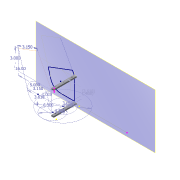
# Autodesk Inventor part: TransferChute
Saved by Autodesk Inventor 2018 (Build 220112000, 112)
## iProperties
Created: 2018-12-12
Part Number: TransferChute
Material: Generic
Document SubType Name: Modeling
Designer: ball
Density: 1 g/cm^3
Appearance: Default
Author: ball
Autodesk Inventor part; units mm, degrees
ref_plane "YZ Plane" through (0, 0, 0) normal (1, 0, 0) x (0, 1, 0)
ref_plane "XZ Plane" through (0, 0, 0) normal (0, 1, 0) x (-1, 0, 0)
sketch "Sketch1" plane through (0, 0, 0) normal (0, 0, 1) x (1, 0, 0)
  line L0 (-8, 88) -> (-8, 100) construction
  line L1 (272, 92) -> (-8, 92) construction
  line L2 (272, 92) -> (-8, 92) construction
  line L3 (-8, 88) -> (-8, 100) construction
  line L4 (-20, 88) -> (-20, 90.5) construction
  line L5 (-8, 88) -> (-20, 88) construction
  line L6 (-20, 88) -> (-20, 8) construction
  line L7 (-20, 88) -> (-147, 88) construction
  line L8 (-147, 88) -> (-147, 164.2) construction
  line L9 (-147, 164.2) -> (-72.1492, 192.4658) construction
  line L10 (-72.1492, 192.4658) -> (-20, 88) construction
  line L11 (-20, 48) -> (-111.8972, 48) construction
  circle A0 centre (-72.0661, 48) radius 40.005 construction
  line L12 (-71.4336, 8) -> (-20, 8) construction
  line L13 (-147, 164.2) -> (-110.5216, 36.974) construction
  point P0 (0, 0)
  dimension "d21" = 80.01
  dimension "d4" = 127
  dimension "d5" = 76.2
  dimension "d6" = 80.01
  dimension "d20" = 91.8972
  dimension "d23" = 15.999
  constraints: 24 end point, 5 horizontal, 4 vertical, 1 coincident, 1 midpoint, 1 point on line, 11 other
  measures "d4" distance of L7.start L7.end
  measures "d5" distance of L7.end L8.end
  measures "d6" distance of L8.end L9.end
  measures "d20" distance of L11.start L11.end
  measures "d23" angle of L8 L13
sketch "Sketch2" plane through (0, 0, 0) normal (0, 1, 0) x (-1, 0, 0)
  line L0 (10.5, -88) -> (20, -88) construction
  circle A0 centre (16, -84) radius 2 construction
  line L1 (16, -84) -> (31.875, -56.5037) construction
  line L2 (16, -84) -> (47.75, -84) construction
  line L3 (20, -88) -> (20, 0) construction
  line L4 (31.875, -56.5037) -> (31.875, -16.4987) construction
  circle A1 centre (31.875, -16.4987) radius 40.005 construction
  circle A2 centre (31.875, -56.5037) radius 40.005 construction
  circle A3 centre (31.875, -56.5037) radius 80.01 construction
  line L5 (111.885, -52.8947) -> (111.885, -78.2947) construction
  point P0 (0, 0)
  dimension "d10" = 31.75
  dimension "d11" = 60
  dimension "d13" = 40.005
  dimension "d14" = 80.01
  dimension "d15" = 80.01
  dimension "d17" = 160.02
  dimension "d18" = 11.875
  dimension "d24" = 25.4
  dimension "d25" = 91.885
  constraints: 12 end point, 4 centre point, 3 coincident, 3 vertical, 2 horizontal, 1 equal length, 1 tangent, 5 other
  measures "d10" distance of L1.start L1.end
  measures "d11" angle of L2 L1
  measures "d13" distance of L1.end L4.end
  measures "d14" diameter of A1
  measures "d15" diameter of A2
  measures "d17" diameter of A3
  measures "d18" distance from line of L3 A1.centre
  measures "d24" distance of L5.start L5.end
  measures "d25" distance from line of L3 L5.end
ref_plane "Work Plane1" through (0, 100, -88) normal (0, 0, -1) x (-1, 0, 0)
sketch "Sketch3" plane through (0, 100, -88) normal (0, 0, -1) x (-1, 0, 0)
  line L0 (10.5, -94.5) -> (20, -94.5) construction
  line L1 (10.5, -9.5) -> (20, -9.5) construction
  line L2 (10.5, -94.5) -> (20, -94.5)
  line L3 (20, -94.5) -> (20, -99.58)
  line L4 (20, -99.58) -> (10.5, -99.58)
  line L5 (10.5, -99.58) -> (10.5, -94.5)
  line L6 (10.5, -9.5) -> (20, -9.5)
  line L7 (20, -9.5) -> (20, -4.42)
  line L8 (20, -4.42) -> (10.5, -4.42)
  line L9 (10.5, -4.42) -> (10.5, -9.5)
  point P0 (0, -100)
  dimension "d26" = 5.08
  dimension "d27" = 5.08
  constraints: 20 end point, 4 horizontal, 4 parallel, 2 perpendicular, 1 point on line, 4 other
  measures "d26" distance of L2.end L3.end
  measures "d27" distance of L7.end L6.end
ref_plane "Work Plane2" through (-20.1567, -4.1567, 0) normal (0, 0, 1) x (1, 0, 0)
extrude "Extrusion1" add sketch "Sketch3" against normal up to surface (88 mm away)
sketch "Sketch4" plane through (0, 100, -88) normal (0, 0, -1) x (-1, 0, 0)
  line L0 (71.4336, -92) -> (20, -92) construction
  line L1 (20, -12) -> (147, -12) construction
  circle A0 centre (72.0661, -52) radius 40.005 construction
  line L2 (20, -92) -> (72.0622, -92.005)
  line L3 (147, 64.2) -> (72.1492, 92.4658) construction
  line L4 (20, -4.42) -> (72.1492, 92.4658) construction
  line L5 (26.6402, 7.9165) -> (120.6802, -27.5957)
  line L6 (147, 64.2) -> (110.5216, -63.026) construction
  line L7 (20, -4.42) -> (26.6402, 7.9165)
  arc A1 (71.4336, -92) -> (110.5216, -63.026) centre (72.0661, -52) ccw
  line L8 (110.5216, -63.026) -> (120.6802, -27.5957)
  line L9 (20, -92) -> (20, -4.42)
  point P0 (0, -100)
  constraints: 13 end point, 3 point on line, 3 tangent, 2 collinear, 2 point on circle, 1 centre point, 1 coincident, 1 parallel, 1 vertical
sketch "Sketch5" plane through (-20, 95.58, -88) normal (0, 1, 0) x (1, 0, 0)
  circle A0 centre (4, -76) radius 2
  circle A1 centre (4, -12) radius 2
  circle A2 centre (4, -44) radius 2
  point P0 (20, -88)
  constraints: 3 centre point, 6 other
extrude "Extrusion2" cut sketch "Sketch5" against normal through all
sketch "Sketch6" plane through (0, 100, -88) normal (0, 0, -1) x (-1, 0, 0)
  point P0 (0, -100)
body "Solid1"
